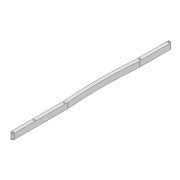
# Autodesk Inventor part: Part_16
Saved by Autodesk Inventor 2022 (Build 260153000, 153)
## iProperties
Created: 2022-05-03
Part Number: Part_16
Material: Generic
Document SubType Name: Modeling
Designer: dell
Density: 1 g/cm^3
Appearance: Default
Author: dell
Autodesk Inventor part; units mm, degrees
ref_plane "YZ Plane" through (0, 0, 0) normal (1, 0, 0) x (0, 1, 0)
ref_plane "XZ Plane" through (0, 0, 0) normal (0, 1, 0) x (-1, 0, 0)
ref_plane "XY Plane" through (0, 0, 0) normal (0, 0, 1) x (1, 0, 0)
sketch "Sketch1" plane through (0, 0, 0) normal (0, 1, 0) x (-1, 0, 0)
  line L0 (0, 0) -> (0, -287.501) construction
  line L1 (-3, 0) -> (-3, -287.501)
  line L2 (3, -287.501) -> (3, 0)
  arc A0 (3, 0) -> (-3, 0) centre (0, 0) ccw
  arc A1 (-3, -287.501) -> (3, -287.501) centre (0, -287.501) ccw
  circle A2 centre (0, 0) radius 1.5
  circle A3 centre (0, -287.501) radius 1.5
  circle A4 centre (0, -39.171) radius 1.5
  circle A5 centre (0, -94.738) radius 1.5
  circle A6 centre (0, -233.822) radius 1.5
  arc A7 (-3, -230.822) -> (-3, -97.738) centre (-800.2278, -164.28) ccw
  arc A8 (3, -230.822) -> (3, -97.738) centre (-794.2278, -164.28) ccw
  point P0 (0, -143.7505)
  dimension "d0" = 6
  dimension "d1" = 287.501
  dimension "d2" = 3
  dimension "d3" = 3
  dimension "d14" = 3
  dimension "d15" = 39.171
  dimension "d16" = 3
  dimension "d17" = 94.738
  dimension "d18" = 3
  dimension "d19" = 233.822
  dimension "d20" = 800
  dimension "d21" = 800
  dimension "d22" = 3
  dimension "d23" = 3
  constraints: 9 centre point, 8 end point, 8 point on circle, 7 point on line, 4 tangent, 2 coincident, 2 horizontal alignment, 1 midpoint, 1 parallel, 1 vertical
  measures "d0" diameter of A1
  measures "d1" distance of L0.end L0.start
  measures "d2" diameter of A2
  measures "d3" diameter of A3
  measures "d14" diameter of A4
  measures "d15" distance of L0.start A4.centre
  measures "d16" diameter of A5
  measures "d17" distance of L0.start A5.centre
  measures "d18" diameter of A6
  measures "d19" distance of L0.start A6.centre
  measures "d20" radius of A7
  measures "d21" radius of A8
  measures "d22" horizontal distance of A6.centre A7.start
  measures "d23" horizontal distance of A5.centre A7.end
extrude "Extrusion1" add sketch "Sketch1" along normal blind 10 contours A0 L2 A1 L1 A7 | A8 L2
body "Solid1"
